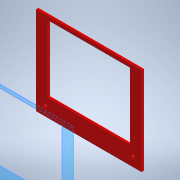
# Autodesk Inventor part: lag3
Saved by Autodesk Inventor 2022 (Build 260153000, 153)
## iProperties
Created: 2023-08-31
Part Number: lag3
Material: Generic
Document SubType Name: Modeling
Designer: THK
Density: 1 g/cm^3
Appearance: Red
Author: THK
Autodesk Inventor part; units mm, degrees
ref_plane "YZ Plane" through (0, 0, 0) normal (1, 0, 0) x (0, 1, 0)
ref_plane "XZ Plane" through (0, 0, 0) normal (0, 1, 0) x (-1, 0, 0)
ref_plane "XY Plane" through (0, 0, 0) normal (0, 0, 1) x (1, 0, 0)
sketch "Sketch1" plane through (0, 0, 0) normal (0, 0, 1) x (1, 0, 0)
  circle A0 centre (-219.1094, -175.8797) radius 11.5 projected
  circle A1 centre (219.1094, -175.8797) radius 11.5 projected
  line L0 (264.1156, -220.8859) -> (-264.1156, -220.8859) projected
  line L1 (264.1156, 220.8859) -> (264.1156, -220.8859) projected
  line L2 (-264.1156, 220.8859) -> (264.1156, 220.8859) projected
  line L3 (-264.1156, -220.8859) -> (-264.1156, 220.8859) projected
  line L4 (200, 196.1016) -> (-200, 196.1016) projected
  line L5 (200, -131.8984) -> (200, 196.1016) projected
  line L6 (-200, -131.8984) -> (200, -131.8984) projected
  line L7 (-200, 196.1016) -> (-200, -131.8984) projected
  line L8 (139, 202.1016) -> (119, 202.1016) projected
  line L9 (206, 187.0016) -> (206, 167.0016) projected
  line L10 (-206, 187.0016) -> (-206, 167.0016) projected
  line L11 (-206, -102.7984) -> (-206, -122.7984) projected
  line L12 (206, -122.7984) -> (206, -102.7984) projected
  line L13 (-206, 202.1016) -> (206, 202.1016)
  line L14 (206, 202.1016) -> (206, -131.8984)
  line L15 (206, -131.8984) -> (-206, -131.8984)
  line L16 (-206, -131.8984) -> (-206, 202.1016)
  line L17 (207, 203.1016) -> (-207, 203.1016)
  line L18 (-207, 203.1016) -> (-207, -132.8984)
  line L19 (-207, -132.8984) -> (207, -132.8984)
  line L20 (207, -132.8984) -> (207, 203.1016)
  circle A2 centre (219.1094, -175.8797) radius 9.5 projected
  circle A3 centre (-219.1094, -175.8797) radius 9.5 projected
  circle A4 centre (-219.1094, -175.8797) radius 11.5 projected
  circle A5 centre (-219.1094, -175.8797) radius 11.5 projected
  circle A6 centre (-219.1094, -175.8797) radius 11.5 projected
  point P0 (0, 0)
  dimension "d0" = 1
  constraints: 16 end point, 4 collinear, 4 parallel, 2 perpendicular, 1 horizontal, 3 other
  measures "d0" distance between parallel lines of L13 L17
extrude "Extrusion1" add sketch "Sketch1" along normal blind 12 contours A0 | A1 | L0 L3 L2 L1
sketch "Sketch2" plane through (0, 0, 0) normal (0, 0, -1) x (-1, 0, 0)
  line L0 (0, 210.8859) -> (254.1156, 210.8859) construction
  line L1 (254.1156, 210.8859) -> (254.1156, 0) construction
  line L2 (254.1156, 0) -> (0, 0) construction
  line L3 (0, 0) -> (0, 210.8859) construction
  line L4 (-264.1156, 220.8859) -> (264.1156, 220.8859) construction
  line L5 (264.1156, 220.8859) -> (264.1156, -220.8859) construction
  point P0 (127.0578, 210.8859)
  point P1 (254.1156, 114.7989)
  dimension "d3" = 10
  dimension "d4" = 10
  constraints: 8 end point, 4 coincident, 2 parallel, 1 horizontal, 1 midpoint, 1 perpendicular, 1 point on line
  measures "d3" distance between parallel lines of L4 L0
  measures "d4" distance between parallel lines of L5 L1
hole "Hole1" at (0, 210.8859, 0) at (-127.0578, 210.8859, 0) at (-254.1156, 210.8859, 0) at (-254.1156, 114.7989, 0) at (-254.1156, 0, 0) direction (0, 0, 1) diameter 2 end through all
mirror "Mirror1" about plane through (0, 0, 0) normal (1, 0, 0) of "Hole1"
mirror "Mirror2" about plane through (0, 0, 0) normal (0, 1, 0) of "Hole1", "Mirror1"
body "Solid1"
